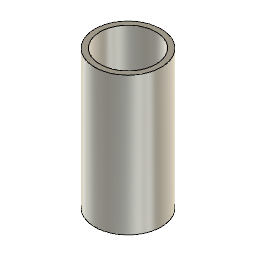
PVCPipeAdapter (Autodesk Fusion 360 design; units mm, degrees)
Autodesk Fusion 360 part; units mm, degrees
sketch "Sketch1" plane through (0, 0, 0) normal (0, 0, 1) x (1, 0, 0)
  circle A0 centre (0, 0) radius 12.954
  circle A1 centre (0, 0) radius 10.922
  dimension "d1" = 25.908
  dimension "d2" = 21.844
  constraint coincident A0.centre A1.centre
  constraint concentric A0 A1
  measures "d1" diameter of A0
  measures "d2" diameter of A1
extrude "Extrude1" add sketch "Sketch1" along normal blind 54
ref_plane "WorkPlane1" through (-12.954, 0, 40.7115) normal (-1, 0, 0) x (0, 1, 0)
sketch "Sketch2" plane through (-12.954, 0, 0) normal (-1, 0, 0) x (0, -1, 0)
  circle A0 centre (0, 18) radius 1.778
  circle A1 centre (0, 36) radius 1.778
  line L0 (0, 18) -> (0, 0) construction
  line L1 (0, 18) -> (0, 36) construction
  line L2 (0, 36) -> (0, 54) construction
  point P0 (0, 54)
  dimension "d6" = 3.556
  dimension "d7" = 3.556
  constraint coincident A0.centre L0.start
  constraint coincident L0.end origin
  constraint vertical L0
  constraint coincident A1.centre L1.end
  constraint parallel L0 L1
  constraint parallel L1 L2
  constraint equal L0 L1
  constraint equal L1 L2
  constraint coincident P0 L2.end
  measures "d6" diameter of A0
  measures "d7" diameter of A1
extrude "Extrude2" cut sketch "Sketch2" along normal up to surface end surface at (10.9084, -0.5444, 36)
